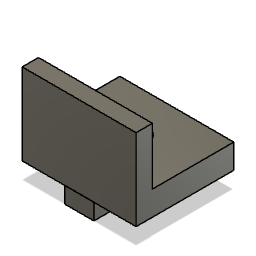
Endstopflag (Autodesk Fusion 360 design; units mm, degrees)
Autodesk Fusion 360 part; units mm, degrees
sketch "Sketch1" plane through (0, 0, 0) normal (0, 1, 0) x (1, 0, 0)
  line L0 (0, 0) -> (0, 10)
  line L1 (0, 0, 0) -> (0, 0, 10)
  line L2 (0, -1, 10) -> (0, 2, 10)
  line L3 (0, 10, 0) -> (0, 10, 3)
  line L4 (0, 10, 3) -> (0, 0, 3)
  line L5 (0, 2, 10) -> (0, 2, 0)
  dimension "d1" = 10
  dimension "d2" = 10
  dimension "d3" = 3
  dimension "d4" = 3
  constraint coincident L0.start origin
  constraint vertical L0
  measures "d1" distance of L0.start L0.end
  measures "d2" distance of L0.start origin
sketch "Sketch1 (curves on the plane with normal 1, 0, 0 at 0 mm)" plane through (0, 0, 0) normal (1, 0, 0) x (0, 0, -1)
  line L0 (0, 0) -> (10, 0)
  line L1 (0, 0) -> (0, 10)
  line L2 (-1, 10) -> (2, 10)
  line L3 (10, 0) -> (10, 3)
  line L4 (10, 3) -> (0, 3)
  line L5 (2, 10) -> (2, 0)
extrude "Extrude1" add sketch "Sketch1 (curves on the plane with normal 1, 0, 0 at 0 mm)" along normal blind 12
sketch "Sketch2" plane through (0, 3, 0) normal (0, 1, 0) x (-1, 0, 0)
  line L0 (0, -10) -> (0, -2)
  line L1 (0, -2) -> (-12, -2)
  line L2 (-12, -2) -> (-12, -10)
  line L3 (-12, -10) -> (0, -10)
  circle A0 centre (-5, -6.5) radius 1.85
  dimension "d7" = 3.7
  measures "d7" diameter of A0
extrude "Extrude2" cut sketch "Sketch2" against normal blind 7 contours A0
move_face "OffsetFaces1" offset 2 1 faces at (0, 1, -4)
move_face "OffsetFaces2" offset 2 1 faces at (7.3333, 2, -10)
sketch "Sketch3" plane through (0, 0, 0) normal (0, -1, 0) x (1, 0, 0)
  circle A0 centre (5, -6.5) radius 1.85
  line L0 (-2, 0) -> (-2, -12)
  line L1 (-2, -12) -> (12, -12)
  line L2 (12, -12) -> (12, 0)
  line L3 (12, 0) -> (-2, 0)
  line L4 (6.7971, -2.669) -> (3.2029, -2.669)
  line L5 (3.2029, -2.669) -> (3.2029, -0.0162)
  line L6 (3.2029, -0.0162) -> (6.7971, -0.0162)
  line L7 (6.7971, -0.0162) -> (6.7971, -2.669)
  line L8 (6.7971, -2.669) -> (3.2029, -0.0162) construction
  line L9 (3.2029, -2.669) -> (6.7971, -0.0162) construction
  point P0 (5, -1.3426)
  constraint horizontal L4
  constraint perpendicular L4 L5
  constraint parallel L4 L6
  constraint parallel L5 L7
  constraint coincident L8 P0
  constraint coincident L9 P0
extrude "Extrude3" add sketch "Sketch3" along normal blind 2 contours L4 L5 L6 L7
